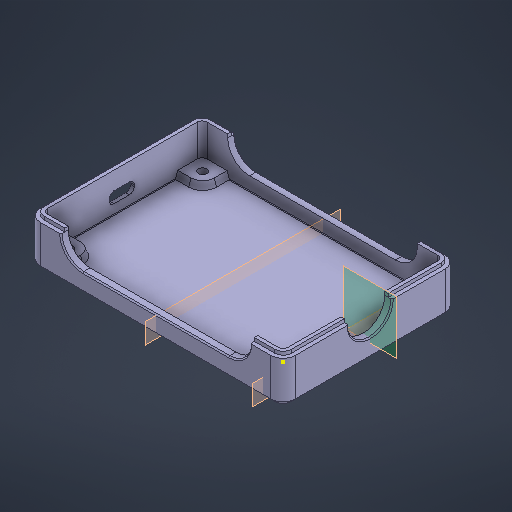
# Autodesk Inventor part: case1
Saved by Autodesk Inventor 2025.2 (Build 292293000, 293)
## iProperties
Created: 2025-10-04
Part Number: case1
Material: Generic
Document SubType Name: Modeling
Designer: micyg
Density: 1 g/cm^3
Appearance: Default
Author: micyg
## iProperties of the stored document case1_3DPrint.ipt
Created: 2025-10-05
Part Number: case1_3DPrint
Material: Generic
Document SubType Name: Modeling
Designer: micyg
Density: 1 g/cm^3
Appearance: Default
Author: micyg
Autodesk Inventor part; units mm, degrees
ref_plane "YZ Plane" through (0, 0, 0) normal (1, 0, 0) x (0, 1, 0)
ref_plane "XZ Plane" through (0, 0, 0) normal (0, 1, 0) x (-1, 0, 0)
ref_plane "XY Plane" through (0, 0, 0) normal (0, 0, 1) x (1, 0, 0)
sketch "Sketch1" plane through (0, 0, 0) normal (0, 1, 0) x (-1, 0, 0)
  line L0 (0, 0) -> (104.9, 0)
  line L1 (104.9, 0) -> (104.9, -71.6)
  line L2 (104.9, -71.6) -> (0, -71.6)
  line L3 (0, -71.6) -> (0, 0)
  line L4 (0, -71.6) -> (104.9, 0) construction
  line L5 (3.45, -3.3) -> (101.45, -3.3) construction
  line L6 (101.45, -3.3) -> (101.45, -68.3) construction
  line L7 (101.45, -68.3) -> (3.45, -68.3) construction
  line L8 (3.45, -68.3) -> (3.45, -3.3) construction
  line L9 (3.45, -3.3) -> (101.45, -68.3) construction
  line L10 (101.45, -3.3) -> (3.45, -68.3) construction
  point P0 (52.45, -35.8)
  dimension "d17" = 98
  dimension "d18" = 65
  dimension "d21" = 71.6
  dimension "d22" = 104.9
  constraints: 22 end point, 4 parallel, 3 midpoint, 2 horizontal, 2 perpendicular
  measures "d17" distance of L6.end L7.end
  measures "d18" distance of L5.end L6.end
  measures "d21" distance between parallel lines of L2 L0
  measures "d22" distance between parallel lines of L3 L1
extrude "Extrusion1" add sketch "Sketch1" along normal blind 17.5
ref_plane "Work Plane7" through (0, 17.5, -35.8) normal (0, 0, -1) x (-1, 0, 0)
fillet "Fillet3" radius 5 4 edges at (-104.9, 8.75, -71.6) (-104.9, 8.75, 0) (0, 8.75, -71.6) (0, 8.75, 0)
chamfer "Chamfer1" distance 2 angle 45 8 edges at (0, 0, -35.8) (-1.4645, 0, -70.1355) (-52.45, 0, -71.6) (-103.4355, 0, -70.1355) (-104.9, 0, -35.8) (-103.4355, 0, -1.4645) (-52.45, 0, 0) (-1.4645, 0, -1.4645)
shell "Shell2" thickness 3 removed faces 1 at (-36.6333, 17.5, -47.7333)
sketch "Sketch2" plane through (-99.9, 3, -68.6) normal (0, 1, 0) x (1, 0, 0)
  line L0 (91.5, -5.3) -> (3.5, -5.3) construction
  line L1 (3.5, -5.3) -> (3.5, -60.3) construction
  line L2 (3.5, -60.3) -> (91.5, -60.3) construction
  line L3 (91.5, -60.3) -> (91.5, -5.3) construction
  arc A0 (91.5, -55.55) -> (86.75, -60.3) centre (91.5, -60.3) ccw
  line L4 (95, 0) -> (0, 0) construction
  arc A1 (-2, -63.6) -> (0, -65.6) centre (0, -63.6) ccw projected
  line L5 (-2, -63.6) -> (-2, -2) projected
  arc A2 (0, 0) -> (-2, -2) centre (0, -2) ccw projected
  line L6 (0, 0) -> (94.9, 0) projected
  arc A3 (96.9, -2) -> (94.9, 0) centre (94.9, -2) ccw projected
  line L7 (96.9, -2) -> (96.9, -63.6) projected
  arc A4 (94.9, -65.6) -> (96.9, -63.6) centre (94.9, -63.6) ccw projected
  line L8 (94.9, -65.6) -> (0, -65.6) projected
  arc A5 (94.9, -68.6) -> (99.9, -63.6) centre (94.9, -63.6) ccw projected
  line L9 (99.9, -63.6) -> (99.9, -2) projected
  arc A6 (99.9, -2) -> (94.9, 3) centre (94.9, -2) ccw projected
  line L10 (94.9, 3) -> (0, 3) projected
  arc A7 (0, 3) -> (-5, -2) centre (0, -2) ccw projected
  line L11 (-5, -2) -> (-5, -63.6) projected
  arc A8 (-5, -63.6) -> (0, -68.6) centre (0, -63.6) ccw projected
  line L12 (0, -68.6) -> (94.9, -68.6) projected
  line L13 (91.5, -55.55) -> (96.9, -55.55)
  line L14 (86.75, -60.3) -> (86.75, -65.6)
  circle A9 centre (91.5, -60.3) radius 1.75
  line L15 (-5, -2) -> (-5, -63.6) projected
  line L16 (-5, -32.8) -> (99.9, -32.8) construction
  line L17 (47.45, -68.6) -> (47.45, 3) construction
  line L18 (3.5, -60.3) -> (91.5, -5.3) construction
  line L19 (47.5, -5.3) -> (47.5, -60.3) construction
  line L20 (-1.5, -0.3) -> (96.5, -0.3) construction
  line L21 (96.5, -0.3) -> (96.5, -65.3) construction
  line L22 (96.5, -65.3) -> (-1.5, -65.3) construction
  line L23 (-1.5, -65.3) -> (-1.5, -0.3) construction
  line L24 (-1.5, -0.3) -> (96.5, -65.3) construction
  arc A10 (86.75, -5.3) -> (91.5, -10.05) centre (91.5, -5.3) ccw
  line L25 (91.5, -10.05) -> (96.9, -10.05)
  line L26 (86.75, -5.3) -> (86.75, 0)
  circle A11 centre (91.5, -5.3) radius 1.75
  arc A12 (8.25, -60.3) -> (3.5, -55.55) centre (3.5, -60.3) ccw
  line L27 (8.25, -60.3) -> (8.25, -65.6)
  circle A13 centre (3.5, -60.3) radius 1.75
  arc A14 (3.5, -10.05) -> (8.25, -5.3) centre (3.5, -5.3) ccw
  line L28 (8.25, -5.3) -> (8.25, 0)
  circle A15 centre (3.5, -5.3) radius 1.75
  line L29 (3.5, -10.05) -> (-2, -10.05)
  line L30 (3.5, -55.55) -> (-2, -55.55)
  point P0 (99.9, -68.6)
  point P1 (47.5, -32.8)
  point P2 (47.5, -32.8)
  point P3 (96.9, -10.05)
  point P4 (8.25, 0)
  point P5 (8.25, -65.6)
  dimension "d13" = 88
  dimension "d14" = 55
  dimension "d25" = 3.5
  dimension "d26" = 3
  dimension "d73" = 65
  dimension "d74" = 98
  dimension "d75" = 0.5
  dimension "d76" = 0.4
  constraints: 42 end point, 16 symmetric about line, 9 midpoint, 9 point on circle, 8 centre point, 7 point on line, 4 parallel, 3 coincident, 3 perpendicular, 3 tangent, 2 horizontal, 6 other
  measures "d13" distance between parallel lines of L1 L3
  measures "d14" distance of L2.end L0.start
  measures "d25" diameter of A9
  measures "d26" radial gap between concentric circles of A0 A9
  measures "d73" distance of L20.end L21.end
  measures "d74" distance of L20.start L20.end
  measures "d75" distance between parallel lines of L5 L23
  measures "d76" distance between parallel lines of L21 L7
extrude "Extrusion2" add sketch "Sketch2" along normal blind 2.75 contours L13 L7 A4 L8 L14 A0 | L25 A10 L26 L6 A3 L7 | L8 A1 L5 L30 A12 L27 | L28 A14 L29 L5 A2 L6
ref_plane "Work Plane1" through (-52.45, 17.5, -3) normal (-1, 0, 0) x (0, -1, 0)
ref_plane "Work Plane2" through (-3, 17.5, -35.8) normal (0, 0, 1) x (1, 0, 0)
ref_plane "Work Plane5" through (-52.4, 3, -35.8) normal (1, 0, 0) x (0, 0, -1)
ref_plane "Work Plane6" through (-8.4, 3, -8.3) normal (1, 0, 0) x (0, 0, -1)
sketch "Sketch12" plane through (-8.4, 3, -8.3) normal (1, 0, 0) x (0, 0, -1)
  line L0 (0, 2.75) -> (-5.3, 2.75) projected
  line L1 (-3.3, 2.75) -> (-5.3, 2.75) projected
  line L2 (4.75, 2.75) -> (-3.3, 2.75) projected
  line L3 (4.75, 2.75) -> (0, 2.75) projected
  line L4 (-1.75, 2.75) -> (1.75, 2.75) projected
  line L5 (-1.75, 2.75) -> (1.75, 2.75) projected
  line L6 (1.75, 0) -> (-1.75, 0) projected
  line L7 (-1.75, 2.75) -> (-1.75, 0) projected
  line L8 (1.75, 2.75) -> (1.75, 0) projected
  line L9 (-8.3, 14.5) -> (-8.3, -1) projected
  line L10 (-8.3, -1) -> (-8.3, 14.5) projected
  line L11 (-1.75, 0) -> (-3, -1.25)
  line L12 (-3, -1.25) -> (-3, -3)
  line L13 (-1.75, 0) -> (0, 0)
  line L14 (-1.75, 0) -> (0, 0)
  line L15 (0, 0) -> (0, -3)
  line L16 (1.75, 0) -> (3, -1.25)
  line L17 (3, -1.25) -> (3, -3)
  line L18 (-6.3, -3) -> (-8.3, -1) projected
  line L19 (-8.3, -1) -> (-3.3, -1) projected
  line L20 (-3.3, -3) -> (-3.3, -1) projected
  line L21 (-3.3, -3) -> (-6.3, -3) projected
  line L22 (-3.3, -3) -> (-3.3, -1) projected
  line L23 (-3.3, -1) -> (58.3, -1) projected
  line L24 (58.3, -3) -> (58.3, -1) projected
  line L25 (58.3, -3) -> (-3.3, -3) projected
  line L26 (-8.3, -1) -> (-3.3, -1) projected
  line L27 (-8.3, -1) -> (-8.3, 14.5) projected
  line L28 (-8.3, 14.5) -> (-3.3, 14.5) projected
  line L29 (-3.3, 14.5) -> (-3.3, -1) projected
  point P0 (-8.3, -3)
  dimension "d77" = 45
  dimension "d78" = 6
  constraints: 14 end point, 3 symmetric about line, 2 point on line, 1 collinear, 1 midpoint, 1 perpendicular
  measures "d77" angle of L12 L11
  measures "d78" distance between parallel lines of L17 L12
revolve "Revolution2" cut sketch "Sketch12" angle 360 about axis through (-8.4, 3, -8.3) along (0, -1, 0) contours L16 L23 L15 L6 | L16 L17 L25 L15 L23
mirror "Mirror6" about plane through (-3, 17.5, -35.8) normal (0, 0, 1) of "Revolution2"
mirror "Mirror7" about plane through (-52.4, 3, -35.8) normal (1, 0, 0) of "Revolution2", "Mirror6"
draft "FaceDraft1" angle 20 pull direction (0, 1, 0) faces at (-13.1367, 4.8333, -8.655) (-13.15, 4.8333, -4.8475) (-4.8809, 4.8333, -13.05) (-13.1367, 3.9167, -62.945) (-4.8809, 4.8333, -58.55) (-13.15, 4.8333, -66.7525) (-96.045, 4.8333, -13.0367) (-99.9858, 4.8333, -13.05) (-91.65, 4.8333, -4.8475) (-94.6646, 4.8333, -58.8783) (-91.65, 4.8333, -66.7525) (-99.9858, 4.8333, -58.55) fixed edges at (-11.7588, 5.75, -11.6588) (-13.15, 5.75, -5.65) (-5.7, 5.75, -13.05) (-11.7588, 5.75, -59.9412) (-5.7, 5.75, -58.55) (-13.15, 5.75, -65.95) (-93.0412, 5.75, -11.6588) (-99.15, 5.75, -13.05) (-91.65, 5.75, -5.65) (-93.0412, 5.75, -59.9412) (-91.65, 5.75, -65.95) (-99.15, 5.75, -58.55)
sketch "Sketch19" plane through (-5, 17.5, -71.6) normal (0, 0, -1) x (-1, 0, 0)
  line L0 (94.9, -15.5) -> (0, -15.5) construction
  line L1 (94.9, 0) -> (94.9, -15.5) construction
  line L2 (0, 0) -> (94.9, 0) construction
  line L3 (0, -15.5) -> (0, 0) construction
  line L4 (47.4, -22.8) -> (47.4, 14.3) construction
  line L5 (8.4, -9) -> (86.4, -9) construction
  line L6 (86.4, -9) -> (86.4, 9)
  line L7 (86.4, 9) -> (8.4, 9)
  line L8 (8.4, 9) -> (8.4, -9)
  line L9 (8.4, -9) -> (86.4, 9) construction
  line L10 (86.4, -9) -> (8.4, 9) construction
  arc A0 (77.4, -9) -> (77.4, 9) centre (77.4, 0) ccw
  arc A1 (17.4, 9) -> (17.4, -9) centre (17.4, 0) ccw
  line L11 (17.4, -9) -> (77.4, -9)
  line L12 (77.4, 9) -> (17.4, 9)
  point P0 (-5, -17.5)
  point P1 (47.4, 0)
  point P2 (86.4, 0)
  point P3 (8.4, 0)
  point P4 (47.4, 0)
  point P5 (47.4, 0)
  dimension "d103" = 78
  dimension "d104" = 9
  constraints: 16 end point, 8 point on line, 5 tangent, 4 midpoint, 4 point on circle, 2 centre point, 2 horizontal, 2 parallel, 1 perpendicular
  measures "d103" distance between parallel lines of L8 L6
  measures "d104" radius of A0
extrude "Extrusion13" cut sketch "Sketch19" against normal up to surface (3 mm away)
mirror "Mirror9" about plane through (0, 17.5, -35.8) normal (0, 0, -1) of "Extrusion13"
sketch "Sketch20" plane through (0, 17.5, -5) normal (1, 0, 0) x (0, 0, -1)
  line L0 (61.6, -15.5) -> (0, -15.5) construction
  line L1 (61.6, 0) -> (61.6, -15.5) construction
  line L2 (0, 0) -> (61.6, 0) construction
  line L3 (0, -15.5) -> (0, 0) construction
  line L4 (30.8, 14.3) -> (30.8, -22.8) construction
  circle A0 centre (30.8, 0) radius 9
  point P0 (-5, -17.5)
  dimension "d109" = 18
  constraints: 1 centre point, 1 midpoint, 1 point on line
  measures "d109" diameter of A0
extrude "Extrusion14" cut sketch "Sketch20" against normal up to surface (3 mm away)
sketch "Sketch21" plane through (-104.9, 17.5, -66.6) normal (-1, 0, 0) x (0, 0, 1)
  line L0 (31.1, -9.65) -> (31.1, -9.85) projected
  line L1 (34.29, -9.85) -> (31.1, -9.85) projected
  arc A0 (34.29, -9.85) -> (35.57, -8.57) centre (34.29, -8.57) ccw projected
  line L2 (35.57, -7.97) -> (35.57, -8.57) projected
  arc A1 (35.57, -7.97) -> (34.29, -6.69) centre (34.29, -7.97) ccw projected
  line L3 (31.1, -6.69) -> (34.29, -6.69) projected
  line L4 (31.1, -6.69) -> (31.1, -6.89) projected
  line L5 (31.1, -6.89) -> (34.29, -6.89) projected
  arc A2 (35.37, -7.97) -> (34.29, -6.89) centre (34.29, -7.97) ccw projected
  line L6 (35.37, -7.97) -> (35.37, -8.57) projected
  arc A3 (34.29, -9.65) -> (35.37, -8.57) centre (34.29, -8.57) ccw projected
  line L7 (34.29, -9.65) -> (31.1, -9.65) projected
  line L8 (31.1, -9.65) -> (31.1, -9.85) projected
  line L9 (27.91, -9.65) -> (31.1, -9.65) projected
  arc A4 (26.83, -8.57) -> (27.91, -9.65) centre (27.91, -8.57) ccw projected
  line L10 (26.83, -7.97) -> (26.83, -8.57) projected
  arc A5 (27.91, -6.89) -> (26.83, -7.97) centre (27.91, -7.97) ccw projected
  line L11 (31.1, -6.89) -> (27.91, -6.89) projected
  line L12 (31.1, -6.69) -> (31.1, -6.89) projected
  line L13 (31.1, -6.69) -> (27.91, -6.69) projected
  arc A6 (27.91, -6.69) -> (26.63, -7.97) centre (27.91, -7.97) ccw projected
  line L14 (26.63, -7.97) -> (26.63, -8.57) projected
  arc A7 (26.63, -8.57) -> (27.91, -9.85) centre (27.91, -8.57) ccw projected
  line L15 (27.91, -9.85) -> (31.1, -9.85) projected
  line L16 (31.1, -5.99) -> (34.29, -5.99)
  arc A8 (36.27, -7.97) -> (34.29, -5.99) centre (34.29, -7.97) ccw
  line L17 (36.27, -7.97) -> (36.27, -8.57)
  arc A9 (34.29, -10.55) -> (36.27, -8.57) centre (34.29, -8.57) ccw
  line L18 (34.29, -10.55) -> (31.1, -10.55)
  line L19 (31.1, -5.99) -> (27.91, -5.99)
  arc A10 (27.91, -5.99) -> (25.93, -7.97) centre (27.91, -7.97) ccw
  line L20 (25.93, -7.97) -> (25.93, -8.57)
  arc A11 (25.93, -8.57) -> (27.91, -10.55) centre (27.91, -8.57) ccw
  line L21 (27.91, -10.55) -> (31.1, -10.55)
  point P0 (66.6, -17.5)
  dimension "d112" = 0.7
  constraints: 12 end point, 8 point on circle, 4 centre point, 8 other
  measures "d112" distance between parallel lines of L16 L3
extrude "Extrusion15" cut sketch "Sketch21" against normal up to surface (3 mm away) contours L7 A3 L6 A2 L5 L4 L3 A1 L2 A0 L1 L0 | L9 A4 L10 A5 L11 L5 A2 L6 A3 L7 | L0 L15 A7 L14 A6 L13 L4 L11 A5 L10 A4 L9 | L16 A8 L17 A9 L18 L21 A11 L20 A10 L19
sketch "Sketch22" plane through (0, 17.5, -35.8) normal (0, 0, -1) x (-1, 0, 0)
  line L0 (101.9, -5.99) -> (101.9, -7.97) projected
  line L1 (104.9, -5.99) -> (101.9, -5.99) projected
  line L2 (104.9, -7.97) -> (104.9, -5.99) projected
  line L3 (104.9, -7.97) -> (101.9, -7.97) projected
  line L4 (101.9, -8.57) -> (101.9, -10.55) projected
  line L5 (104.9, -8.57) -> (101.9, -8.57) projected
  line L6 (104.9, -10.55) -> (104.9, -8.57) projected
  line L7 (104.9, -10.55) -> (101.9, -10.55) projected
  line L8 (101.9, -7.97) -> (101.9, -8.57) projected
  line L9 (104.9, -7.97) -> (101.9, -7.97) projected
  line L10 (104.9, -8.57) -> (104.9, -7.97) projected
  line L11 (104.9, -8.57) -> (101.9, -8.57) projected
  line L12 (104.9, -5.99) -> (101.9, -5.99) projected
  line L13 (104.9, -5.99) -> (101.9, -5.99) projected
  line L14 (104.9, -10.55) -> (101.9, -10.55) projected
  line L15 (104.9, -10.55) -> (101.9, -10.55) projected
  line L16 (104.9, -5.99) -> (104.9, -7.97) projected
  line L17 (104.9, -7.97) -> (104.9, -8.57) projected
  line L18 (104.9, -8.57) -> (104.9, -10.55) projected
  line L19 (104.9, -10.55) -> (104.9, -8.57) projected
  line L20 (104.9, -8.57) -> (104.9, -7.97) projected
  line L21 (104.9, -7.97) -> (104.9, -5.99) projected
  line L22 (104.9, 0) -> (104.9, -15.5) projected
  line L23 (104.9, -15.5) -> (104.9, 0) projected
  line L24 (103.4, -10.55) -> (103.4, -11.85)
  line L25 (103.4, -11.85) -> (104.9, -13.1086)
  point P0 (0, -17.5)
  point P1 (103.4, -10.55)
  dimension "d116" = 50
  dimension "d123" = 1.3
  constraints: 4 end point, 1 midpoint, 1 point on line, 1 vertical
  measures "d116" angle of L24 L25
  measures "d123" distance from line of L7 L24.end
sketch3d "3D Sketch3"
  line L0 (-104.9, 6.95, -38.69) -> (-104.9, 6.95, -32.31)
  arc A0 (-104.9, 6.95, -32.31) -> (-104.9, 8.93, -30.33) centre (-104.9, 8.93, -32.31) ccw
  line L1 (-104.9, 8.93, -30.33) -> (-104.9, 9.53, -30.33)
  arc A1 (-104.9, 9.53, -30.33) -> (-104.9, 11.51, -32.31) centre (-104.9, 9.53, -32.31) ccw
  line L2 (-104.9, 11.51, -32.31) -> (-104.9, 11.51, -38.69)
  arc A2 (-104.9, 11.51, -38.69) -> (-104.9, 9.53, -40.67) centre (-104.9, 9.53, -38.69) ccw
  line L3 (-104.9, 9.53, -40.67) -> (-104.9, 8.93, -40.67)
  arc A3 (-104.9, 8.93, -40.67) -> (-104.9, 6.95, -38.69) centre (-104.9, 8.93, -38.69) ccw
sweep "Sweep2" cut profiles "Sketch22" path "3D Sketch3" contours L22 L25 L24 L7
sketch "Sketch23" plane through (0, 17.5, 0) normal (0, 1, 0) x (1, 0, 0)
  point P0 (0, 0)
sketch "Sketch24" plane through (0, 17.5, 0) normal (0, 1, 0) x (1, 0, 0)
  line L0 (-91.4, 0) -> (-91.4, 3) projected
  line L1 (-91.4, 3) -> (-99.9, 3) projected
  arc A0 (-101.9, 5) -> (-99.9, 3) centre (-99.9, 5) ccw projected
  line L2 (-101.9, 5) -> (-101.9, 66.6) projected
  arc A1 (-99.9, 68.6) -> (-101.9, 66.6) centre (-99.9, 66.6) ccw projected
  line L3 (-99.9, 68.6) -> (-91.4, 68.6) projected
  line L4 (-91.4, 68.6) -> (-91.4, 71.6) projected
  line L5 (-91.4, 71.6) -> (-99.9, 71.6) projected
  arc A2 (-99.9, 71.6) -> (-104.9, 66.6) centre (-99.9, 66.6) ccw projected
  line L6 (-104.9, 66.6) -> (-104.9, 5) projected
  arc A3 (-104.9, 5) -> (-99.9, 0) centre (-99.9, 5) ccw projected
  line L7 (-99.9, 0) -> (-91.4, 0) projected
  line L8 (-3, 44.8) -> (0, 44.8) projected
  line L9 (0, 44.8) -> (0, 66.6) projected
  arc A4 (0, 66.6) -> (-5, 71.6) centre (-5, 66.6) ccw projected
  line L10 (-5, 71.6) -> (-13.4, 71.6) projected
  line L11 (-13.4, 71.6) -> (-13.4, 68.6) projected
  line L12 (-13.4, 68.6) -> (-5, 68.6) projected
  arc A5 (-3, 66.6) -> (-5, 68.6) centre (-5, 66.6) ccw projected
  line L13 (-3, 66.6) -> (-3, 44.8) projected
  line L14 (0, 26.8) -> (-3, 26.8) projected
  line L15 (-3, 26.8) -> (-3, 5) projected
  arc A6 (-5, 3) -> (-3, 5) centre (-5, 5) ccw projected
  line L16 (-5, 3) -> (-13.4, 3) projected
  line L17 (-13.4, 3) -> (-13.4, 0) projected
  line L18 (-13.4, 0) -> (-5, 0) projected
  arc A7 (-5, 0) -> (0, 5) centre (-5, 5) ccw projected
  line L19 (0, 5) -> (0, 26.8) projected
  line L20 (-3, 44.8) -> (0, 44.8) projected
  line L21 (-3, 26.8) -> (-3, 44.8) projected
  line L22 (0, 26.8) -> (-3, 26.8) projected
  line L23 (0, 44.8) -> (0, 26.8) projected
  line L24 (-13.4, 71.6) -> (-13.4, 68.6) projected
  line L25 (-1.6, 66.6) -> (-1.6, 5)
  line L26 (0, 5) -> (0, 26.8) projected
  arc A8 (-5, 1.6) -> (-1.6, 5) centre (-5, 5) ccw
  arc A9 (-5, 3) -> (-3, 5) centre (-5, 5) ccw projected
  line L27 (-13.4, 1.6) -> (-5, 1.6)
  arc A10 (-1.6, 66.6) -> (-5, 70) centre (-5, 66.6) ccw
  line L28 (-5, 70) -> (-13.4, 70)
  arc A11 (-3, 66.6) -> (-5, 68.6) centre (-5, 66.6) ccw projected
  line L29 (-91.4, 68.6) -> (-91.4, 71.6) projected
  line L30 (-91.4, 70) -> (-99.9, 70)
  line L31 (-103.3, 66.6) -> (-103.3, 5)
  line L32 (-99.9, 1.6) -> (-91.4, 1.6)
  arc A12 (-103.3, 5) -> (-99.9, 1.6) centre (-99.9, 5) ccw
  arc A13 (-99.9, 70) -> (-103.3, 66.6) centre (-99.9, 66.6) ccw
  point P0 (0, 0)
  point P1 (-1.6, 26.8)
  point P2 (-1.6, 44.8)
  dimension "d119" = 1.4
  dimension "d120" = 1.4
  constraints: 12 end point, 8 point on circle, 8 tangent, 6 parallel, 4 centre point, 4 concentric, 4 point on line
  measures "d119" distance between parallel lines of L15 L25
  measures "d120" distance between parallel lines of L1 L32
extrude "Extrusion16" add sketch "Sketch24" along normal blind 1.4 contours L32 A12 L31 A13 L30 L4 L3 A1 L2 A0 L1 L0 | L13 A5 L12 L11 L28 A10 L25 L8 | L14 L25 A8 L27 L17 L16 A6 L15
chamfer "Chamfer2" distance 0.5 angle 45 7 edges at (-16.036, 11.136, -71.6) (-52.4, 8.5, -71.6) (-88.764, 11.136, -71.6) (-88.764, 11.136, 0) (-52.4, 8.5, 0) (-16.036, 11.136, 0) (0, 8.5, -35.8)
body "Solid1"
